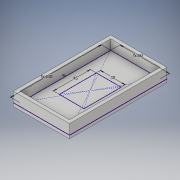
# Autodesk Inventor part: parametric cup
Saved by Autodesk Inventor 2019.3 (Build 233278000, 278)
## iProperties
Created: 2019-07-22
Part Number: parametric cup
Material: Generic
Document SubType Name: Modeling
Designer: Frienddo
Density: 1 g/cm^3
Appearance: Default
Author: Frienddo
Autodesk Inventor part; units mm, degrees
ref_plane "YZ Plane" through (0, 0, 0) normal (1, 0, 0) x (0, 1, 0)
ref_plane "XZ Plane" through (0, 0, 0) normal (0, 1, 0) x (-1, 0, 0)
ref_plane "XY Plane" through (0, 0, 0) normal (0, 0, 1) x (1, 0, 0)
sketch "Sketch1" plane through (0, 0, 0) normal (0, 1, 0) x (-1, 0, 0)
  line L0 (-30, 55) -> (30, 55)
  line L1 (30, 55) -> (30, -55)
  line L2 (30, -55) -> (-30, -55)
  line L3 (-30, -55) -> (-30, 55)
  line L4 (-30, 55) -> (30, -55) construction
  line L5 (30, 55) -> (-30, -55) construction
  line L6 (34, -59) -> (34, 59)
  line L7 (34, 59) -> (-34, 59)
  line L8 (-34, 59) -> (-34, -59)
  line L9 (-34, -59) -> (34, -59)
  line L10 (-15, 22.5) -> (15, 22.5)
  line L11 (15, 22.5) -> (15, -22.5)
  line L12 (15, -22.5) -> (-15, -22.5)
  line L13 (-15, -22.5) -> (-15, 22.5)
  line L14 (-15, 22.5) -> (15, -22.5) construction
  line L15 (15, 22.5) -> (-15, -22.5) construction
  point P0 (0, 0)
  dimension "d0" = 60
  dimension "d1" = 110
  dimension "d2" = 4
  dimension "d7" = 30
  dimension "d8" = 45
  constraints: 32 end point, 6 parallel, 4 midpoint, 3 perpendicular, 2 horizontal, 3 other
  measures "d0" distance of L1.end L2.end
  measures "d1" distance of L0.end L1.end
  measures "d2" distance between parallel lines of L1 L6
  measures "d7" distance of L11.end L12.end
  measures "d8" distance of L10.end L11.end
extrude "Extrusion1" add sketch "Sketch1" along normal blind 12 contours L9 L8 L7 L6
extrude "Extrusion2" add sketch "Sketch1" against normal blind 4 contours L0 L1 L2 L3 | L9 L8 L7 L6 | L10 L11 L12 L13
extrude "Extrusion3" add sketch "Sketch1" against normal blind 19 contours L10 L11 L12 L13
chamfer "Chamfer1" distance 10 angle 45 4 edges at (0, -4, 22.5) (15, -4, 0) (0, -4, -22.5) (-15, -4, 0)
sketch "Sketch3" plane through (0, 0, 0) normal (1, 0, 0) x (0, 1, 0)
  line L0 (-19, -22.5) -> (-19, 22.5) projected
  line L1 (-19, -12.2) -> (-11.5, -12.2)
  line L2 (-11.5, -12.2) -> (-11.5, -17.8)
  line L3 (-11.5, -17.8) -> (-19, -17.8)
  line L4 (-19, -17.8) -> (-19, -12.2)
  arc A0 (-11.5, -17.8) -> (-11.5, -12.2) centre (-11.5, -15) ccw
  line L5 (-19, -2.2) -> (-11.5, -2.2)
  line L6 (-11.5, -2.2) -> (-11.5, -7.8)
  line L7 (-11.5, -7.8) -> (-19, -7.8)
  line L8 (-19, -7.8) -> (-19, -2.2)
  arc A1 (-11.5, -7.8) -> (-11.5, -2.2) centre (-11.5, -5) ccw
  line L9 (-19, 7.8) -> (-11.5, 7.8)
  line L10 (-11.5, 7.8) -> (-11.5, 2.2)
  line L11 (-11.5, 2.2) -> (-19, 2.2)
  line L12 (-19, 2.2) -> (-19, 7.8)
  arc A2 (-11.5, 2.2) -> (-11.5, 7.8) centre (-11.5, 5) ccw
  line L13 (-19, 17.8) -> (-11.5, 17.8)
  line L14 (-11.5, 17.8) -> (-11.5, 12.2)
  line L15 (-11.5, 12.2) -> (-19, 12.2)
  line L16 (-19, 12.2) -> (-19, 17.8)
  arc A3 (-11.5, 12.2) -> (-11.5, 17.8) centre (-11.5, 15) ccw
  line L17 (-19, 2.2) -> (-19, -2.2) construction
  point P0 (0, 0)
  point P1 (-19, 0)
  point P2 (-19, 0)
  dimension "d14" = 7.5
  dimension "d15" = 5.6
  dimension "d18" = 10
  constraints: 34 end point, 8 point on circle, 4 centre point, 4 midpoint, 2 parallel, 2 vertical, 1 horizontal, 1 perpendicular, 1 point on line, 30 other
  measures "d14" distance of L2.end L3.end
  measures "d15" distance of L1.end L2.end
  measures "d18" distance of L1.start L5.start
extrude "Extrusion4" cut sketch "Sketch3" along normal mid plane 20.6
equation "\"d0\" = wid"
equation "\"d1\" = len"
equation "\"d3\" = hei"
equation "\"len\" = 110"
equation "\"wid\" = 60"
equation "\"hei\" = 12"
body "Solid1"
